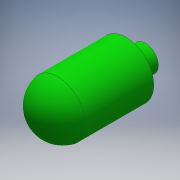
# Autodesk Inventor part: pie
Saved by Autodesk Inventor 2016 (Build 200138000, 138)
## iProperties
Created: 2016-02-19
Part Number: pie
Material: Genérico
Document SubType Name: Modeling
Designer: Usuario1
Density: 1 g/cm^3
Appearance: Valor por defecto
Author: Usuario1
Autodesk Inventor part; units mm, degrees
ref_plane "YZ Plane" through (0, 0, 0) normal (1, 0, 0) x (0, 1, 0)
ref_plane "XZ Plane" through (0, 0, 0) normal (0, 1, 0) x (-1, 0, 0)
ref_plane "XY Plane" through (0, 0, 0) normal (0, 0, 1) x (1, 0, 0)
sketch "Boceto1" plane through (0, 0, 0) normal (0, 0, 1) x (1, 0, 0)
  line L0 (-1.2847, 1.0744) -> (-1.2847, 4.2338)
  line L1 (-0.9847, 1.1029) -> (-0.9847, 3.9338)
  arc A0 (-1.2847, 1.0744) -> (0, 0) centre (0, 1.3052) ccw
  arc A1 (-0.9847, 1.1029) -> (0, 0.3) centre (0, 1.3052) ccw
  line L2 (0, 3.9338) -> (-0.9847, 3.9338)
  line L3 (0, 0) -> (0, 4.5338)
  line L4 (-0.6, 4.5338) -> (-0.6, 4.2338)
  line L5 (-0.6, 4.5338) -> (0, 4.5338)
  line L6 (0, 0.3) -> (0, 0)
  line L7 (-1.2847, 4.2338) -> (-0.6, 4.2338)
  line L8 (0, 4.5338) -> (0, 3.9338)
  line L9 (0, 4.5338) -> (0, 3.9338)
  line L10 (0, 3.9338) -> (-0.9847, 3.9338)
  line L11 (-0.9847, 3.9338) -> (-0.9847, 1.1029)
  point P0 (0, 0)
  constraints: 24 end point, 4 point on circle, 2 centre point, 2 point on line, 1 perpendicular, 1 vertical
revolve "Revolución1" add sketch "Boceto1" angle 360 about axis through (0, 0, 0) along (0, 1, 0) contours L0 L7 L4 L5 L3 L2 L1 A1 A0
sketch "Boceto2" plane through (0, 4.5338, 0) normal (0, 1, 0) x (1, 0, 0)
  circle A0 centre (0, 0) radius 0.6 projected
  point P0 (0, 0)
extrude "Extrusión1" add sketch "Boceto2" along normal blind 0.6
